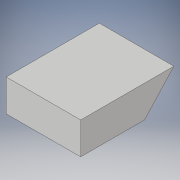
# Autodesk Inventor part: SouthWestWallBlockAngle
Saved by Autodesk Inventor 2018 (Build 220112000, 112)
## iProperties
Created: 2019-04-28
Part Number: SouthWestWallBlockAngle
Material: Generic
Document SubType Name: Modeling
Designer: snipe
Density: 1 g/cm^3
Appearance: Default
Author: snipe
Autodesk Inventor part; units mm, degrees
ref_plane "YZ Plane" through (0, 0, 0) normal (1, 0, 0) x (0, 1, 0)
ref_plane "XY Plane" through (0, 0, 0) normal (0, 0, 1) x (1, 0, 0)
sketch "Sketch1" plane through (0, 0, 0) normal (0, 1, 0) x (-1, 0, 0)
  line L0 (711.2, 609.6) -> (-711.2, 609.6)
  line L1 (-711.2, 609.6) -> (-711.2, -609.6)
  line L2 (-711.2, -609.6) -> (711.2, -609.6)
  line L3 (711.2, -609.6) -> (711.2, 609.6)
  line L4 (0, -853.44) -> (0, 853.44) projected
  line L5 (-995.68, 0) -> (995.68, 0) projected
  line L6 (995.68, 0) -> (-995.68, 0) projected
  line L7 (0, -853.44) -> (0, 853.44) projected
  point P0 (0, 0)
  dimension "d0" = 1422.4
  dimension "d1" = 1219.2
  constraints: 8 end point, 2 parallel, 1 horizontal, 1 perpendicular, 2 other
  measures "d0" distance of L2.end L1.end
  measures "d1" distance of L1.end L0.end
ref_plane "Work Plane1" through (0, 609.6, 0) normal (0, 1, 0) x (-1, 0, 0)
sketch "Sketch2" plane through (0, 609.6, 0) normal (0, 1, 0) x (-1, 0, 0)
  line L0 (711.2, -609.6) -> (711.2, 609.6) projected
  line L1 (711.2, 609.6) -> (-711.2, 609.6) projected
  line L2 (-711.2, 609.6) -> (-711.2, -609.6) projected
  line L3 (711.2, 609.6) -> (-711.2, 609.6)
  line L4 (-711.2, 609.6) -> (-711.2, -609.6)
  line L5 (711.2, -609.6) -> (711.2, 609.6)
  line L6 (711.2, -609.6) -> (711.2, -1168.4)
  line L7 (711.2, -1168.4) -> (-711.2, -1168.4)
  line L8 (-711.2, -1168.4) -> (-711.2, -609.6)
  line L9 (711.2, -1168.4) -> (-711.2, -1168.4)
  line L10 (-711.2, -1168.4) -> (-711.2, 609.6)
  line L11 (-711.2, 609.6) -> (711.2, 609.6)
  line L12 (711.2, 609.6) -> (711.2, -1168.4)
  line L13 (-711.2, 609.6) -> (711.2, 609.6)
  line L14 (711.2, 609.6) -> (711.2, -1168.4)
  line L15 (711.2, -1168.4) -> (-711.2, -1168.4)
  line L16 (-711.2, -1168.4) -> (-711.2, 609.6)
  point P0 (0, 0)
  dimension "d3" = 1422.4
  dimension "d4" = 558.8
  constraints: 28 end point, 6 parallel, 3 horizontal, 3 perpendicular
  measures "d3" distance of L6.end L7.end
  measures "d4" distance of L6.start L6.end
loft "Loft1" add profiles "Sketch1", "Sketch2"
body "Solid1"
